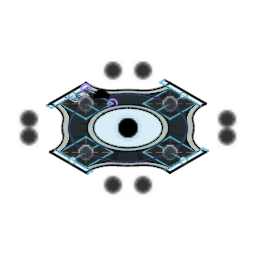
_Round About - Ruby.f2236e12-3166-4e72-b55a-dd2a6dc33c33 (Autodesk Fusion 360 design; units mm, degrees)
Autodesk Fusion 360 part; units mm, degrees
sketch "Sketch1" plane through (0, 0, 0) normal (0, 0, 1) x (1, 0, 0)
  circle A0 centre (0, 0) radius 660.4
  line L0 (660.4, 0) -> (1270, 0)
  line L1 (0, -660.4) -> (0, -1270)
  line L2 (-660.4, 0) -> (-1269.999981, 0)
  line L3 (0, 660.4) -> (0, 1270)
  circle A1 centre (0, 0) radius 965.2
  line L4 (1269.999981, 304.8) -> (660.400019, 304.8)
  line L5 (660.400019, 304.8) -> (660.400019, -304.8)
  line L6 (660.400019, -304.8) -> (1269.999981, -304.8)
  line L7 (1269.999981, -304.8) -> (1269.999981, 304.8)
  line L8 (1269.999981, 304.8) -> (660.400019, -304.8) construction
  line L9 (660.400019, 304.8) -> (1269.999981, -304.8) construction
  line L10 (304.8, 1270) -> (-304.8, 1270)
  line L11 (-304.8, 1270) -> (-304.8, 660.4)
  line L12 (-304.8, 660.4) -> (304.8, 660.4)
  line L13 (304.8, 660.4) -> (304.8, 1270)
  line L14 (304.8, 1270) -> (-304.8, 660.4) construction
  line L15 (-304.8, 1270) -> (304.8, 660.4) construction
  line L16 (-660.39999, 304.8) -> (-1269.99999, 304.8)
  line L17 (-1269.99999, 304.8) -> (-1269.99999, -304.8)
  line L18 (-1269.99999, -304.8) -> (-660.39999, -304.8)
  line L19 (-660.39999, -304.8) -> (-660.39999, 304.8)
  line L20 (-660.39999, 304.8) -> (-1269.99999, -304.8) construction
  line L21 (-1269.99999, 304.8) -> (-660.39999, -304.8) construction
  line L22 (304.8, -660.4) -> (-304.8, -660.4)
  line L23 (-304.8, -660.4) -> (-304.8, -1270)
  line L24 (-304.8, -1270) -> (304.8, -1270)
  line L25 (304.8, -1270) -> (304.8, -660.4)
  line L26 (304.8, -660.4) -> (-304.8, -1270) construction
  line L27 (-304.8, -660.4) -> (304.8, -1270) construction
  point P0 (965.2, 0)
  point P1 (0, 965.2)
  point P2 (-965.19999, 0)
  point P3 (0, -965.2)
  dimension "d1" = 1320.8
  dimension "d2" = 609.6
  dimension "d3" = 609.6
  dimension "d4" = 609.6
  dimension "d5" = 304.8
  dimension "d6" = 609.6
  dimension "d7" = 609.6
  dimension "d8" = 609.6
  dimension "d9" = 609.6
  dimension "d10" = 609.6
  dimension "d11" = 609.6
  dimension "d12" = 609.6
  constraint coincident A0.centre A1.centre
  constraint coincident A0 L0.start
  constraint horizontal L0
  constraint coincident A0 L1.start
  constraint vertical L1
  constraint coincident A0 L2.start
  constraint horizontal L2
  constraint coincident A0 L3.start
  constraint vertical L3
  constraint horizontal L4
  constraint perpendicular L4 L5
  constraint parallel L4 L6
  constraint parallel L5 L7
  constraint coincident L8 P0
  constraint coincident L9 P0
  constraint midpoint L0 P0
  constraint horizontal L10
  constraint perpendicular L10 L11
  constraint parallel L10 L12
  constraint parallel L11 L13
  constraint coincident L14 P1
  constraint coincident L15 P1
  constraint midpoint L3 P1
  constraint horizontal L16
  constraint perpendicular L16 L17
  constraint parallel L16 L18
  constraint parallel L17 L19
  constraint horizontal L22
  constraint perpendicular L22 L23
  constraint parallel L22 L24
  constraint parallel L23 L25
  constraint coincident L26 P3
  constraint coincident L27 P3
  constraint midpoint L1 P3
  measures "d1" diameter of A0
  measures "d2" distance of L0.start L0.end
  measures "d3" distance of L1.start L1.end
  measures "d4" distance of L3.start L3.end
  measures "d7" distance of L11.end L12.end
  measures "d8" distance of L10.end L11.end
  measures "d11" distance of L23.end L24.end
  measures "d12" distance of L22.end L23.end
extrude "Extrude1" add sketch "Sketch1" along normal blind 6.35 contours A0 A1 L5 L6 L22 L25 | L0 A1 L4 L5 | A0 A1 L4 L5 L12 L13 | L0 A1 L5 L6 | L3 A1 L11 L12 | A0 A1 L11 L12 L16 L19 | L3 A1 L12 L13 | A0 A1 L18 L19 L22 L23 | L1 A1 L22 L25 | L1 A1 L22 L23 | L2 A1 L18 L19 | L2 A1 L16 L19 picked at (676.405382, -534.145656) picked at (754.647884, 169.987105) picked at (676.405382, 534.145656) picked at (754.647877, -169.987105) picked at (-169.987105, 754.647871) picked at (-676.405382, 534.145656) picked at (169.987105, 754.647871) picked at (-676.405382, -534.145656) picked at (169.987105, -754.647871) picked at (-169.987105, -754.647871) picked at (-754.647865, -169.987105) picked at (-754.647868, 169.987105) makes body 1
extrude "Extrude2" add sketch "Sketch1" along normal blind 6.35 contours L0 A1 L4 L7 | L0 A1 L6 L7 | L3 A1 L10 L11 | L3 A1 L10 L13 | L1 A1 L24 L25 | L1 A1 L23 L24 | L2 A1 L17 L18 | L2 A1 L16 L17 picked at (1166.556681, 135.990587) picked at (1166.556675, -135.990587) picked at (-135.990587, 1166.556687) picked at (135.990587, 1166.556687) picked at (135.990587, -1166.556687) picked at (-135.990587, -1166.556687) picked at (-1166.556678, -135.990587) picked at (-1166.556681, 135.990587) bodies 1
fillet "Fillet1" radius 660.4 1 edges at (-915.810024, -304.8, 3.175) on bodies 1
fillet "Fillet2" radius 660.4 1 edges at (-304.8, -915.810024, 3.175) on bodies 1
fillet "Fillet3" radius 660.4 1 edges at (304.8, -915.810024, 3.175) on bodies 1
fillet "Fillet4" radius 660.4 1 edges at (915.810024, -304.8, 3.175) on bodies 1
fillet "Fillet5" radius 660.4 1 edges at (915.810024, 304.8, 3.175) on bodies 1
fillet "Fillet6" radius 660.4 1 edges at (304.8, 915.810024, 3.175) on bodies 1
fillet "Fillet7" radius 660.4 1 edges at (-304.8, 915.810024, 3.175) on bodies 1
fillet "Fillet8" radius 660.4 1 edges at (-915.810024, 304.8, 3.175) on bodies 1
sketch "Sketch2" plane through (0, 0, 6.35) normal (0, 0, 1) x (-1, 0, 0)
  arc A0 (572.40726, -777.149258) -> (777.149258, -572.40726) centre (0, 0) ccw
  arc A1 (1269.99999, -304.8) -> (777.149258, -572.40726) centre (1308.882961, -964.054332) ccw
  line L0 (1269.99999, -304.8) -> (1269.99999, 304.8)
  arc A2 (777.149258, 572.40726) -> (1269.99999, 304.8) centre (1308.882961, 964.054332) ccw
  arc A3 (777.149258, 572.40726) -> (572.40726, 777.149258) centre (0, 0) ccw
  arc A4 (304.8, 1270) -> (572.40726, 777.149258) centre (964.054333, 1308.88296) ccw
  line L1 (304.8, 1270) -> (-304.8, 1270)
  arc A5 (-572.40726, 777.149258) -> (-304.8, 1270) centre (-964.054333, 1308.88296) ccw
  arc A6 (-572.40726, 777.149258) -> (-777.149258, 572.407259) centre (0, 0) ccw
  arc A7 (-1269.999981, 304.8) -> (-777.149258, 572.407259) centre (-1308.882961, 964.054332) ccw
  line L2 (-1269.999981, 304.8) -> (-1269.999981, -304.8)
  arc A8 (-777.149258, -572.407259) -> (-1269.999981, -304.8) centre (-1308.882961, -964.054332) ccw
  arc A9 (-777.149258, -572.407259) -> (-572.40726, -777.149258) centre (0, 0) ccw
  arc A10 (-304.8, -1270) -> (-572.40726, -777.149258) centre (-964.054333, -1308.88296) ccw
  line L3 (-304.8, -1270) -> (304.8, -1270)
  arc A11 (572.40726, -777.149258) -> (304.8, -1270) centre (964.054333, -1308.88296) ccw
  arc A12 (660.4, 0) -> (660.399997, -0.064797) centre (0, 0) ccw
  line L4 (660.4, 0) -> (660.399997, -0.064797)
  line L5 (558.8, 0.002492) -> (558.799997, -0.057321)
  arc A13 (558.8, 0.002492) -> (558.799997, -0.057321) centre (0, 0) ccw
  line L6 (-1371.599981, 408.785014) -> (-1371.599981, -408.785014)
  arc A14 (-858.954443, -632.660655) -> (-1371.599981, -408.785014) centre (-1308.882961, -964.054332) ccw
  arc A15 (-858.954443, -632.660655) -> (-632.660656, -858.954443) centre (0, 0) ccw
  arc A16 (-408.785017, -1371.6) -> (-632.660656, -858.954443) centre (-964.054333, -1308.88296) ccw
  line L7 (-408.785017, -1371.6) -> (408.785017, -1371.6)
  arc A17 (632.660656, -858.954443) -> (408.785017, -1371.6) centre (964.054333, -1308.88296) ccw
  arc A18 (632.660656, -858.954443) -> (858.954443, -632.660656) centre (0, 0) ccw
  arc A19 (1371.59999, -408.785016) -> (858.954443, -632.660656) centre (1308.882961, -964.054332) ccw
  line L8 (1371.59999, -408.785016) -> (1371.59999, 408.785016)
  arc A20 (858.954443, 632.660656) -> (1371.59999, 408.785016) centre (1308.882961, 964.054332) ccw
  arc A21 (858.954443, 632.660656) -> (632.660656, 858.954443) centre (0, 0) ccw
  arc A22 (408.785017, 1371.6) -> (632.660656, 858.954443) centre (964.054333, 1308.88296) ccw
  line L9 (408.785017, 1371.6) -> (-408.785017, 1371.6)
  arc A23 (-632.660656, 858.954443) -> (-408.785017, 1371.6) centre (-964.054333, 1308.88296) ccw
  arc A24 (-632.660656, 858.954443) -> (-858.954443, 632.660655) centre (0, 0) ccw
  arc A25 (-1371.599981, 408.785014) -> (-858.954443, 632.660655) centre (-1308.882961, 964.054332) ccw
  line L10 (-1371.599981, 408.785014) -> (-1269.999981, 408.785014)
  line L11 (-1269.999981, 408.785014) -> (-1269.999981, -457.199993)
  line L12 (-1269.999981, -457.199993) -> (-1371.599981, -457.199993)
  line L13 (-1371.599981, -457.199993) -> (-1371.599981, 408.785014)
  line L14 (-408.785017, -1371.6) -> (533.399992, -1371.6)
  line L15 (533.399992, -1371.6) -> (533.399992, -1269.999981)
  line L16 (533.399992, -1269.999981) -> (-408.785017, -1269.999981)
  line L17 (-408.785017, -1269.999981) -> (-408.785017, -1371.6)
  line L18 (1371.59999, -408.785016) -> (1269.999981, -408.785016)
  line L19 (1269.999981, -408.785016) -> (1269.999981, 482.599993)
  line L20 (1269.999981, 482.599993) -> (1371.59999, 482.599993)
  line L21 (1371.59999, 482.599993) -> (1371.59999, -408.785016)
  line L22 (408.785017, 1371.6) -> (-447.666394, 1371.6)
  line L23 (-447.666394, 1371.6) -> (-447.666394, 1270)
  line L24 (-447.666394, 1270) -> (408.785017, 1270)
  line L25 (408.785017, 1270) -> (408.785017, 1371.6)
  line L26 (660.39999, -304.8, -6.35) -> (1269.99999, -304.8, -6.35)
  circle A26 through (965.2, 0, -6.35) (-482.6, 835.88772, -6.35) (-482.6, -835.88772, -6.35)
  point P0 (915.810024, -304.8)
  dimension "d33" = -101.6
  dimension "d34" = -101.6
  constraint horizontal L10
  constraint vertical L11
  constraint horizontal L12
  constraint vertical L13
  constraint horizontal L14
  constraint vertical L15
  constraint horizontal L16
  constraint vertical L17
  constraint horizontal L18
  constraint vertical L19
  constraint horizontal L20
  constraint vertical L21
  constraint horizontal L22
  constraint vertical L23
  constraint horizontal L24
  constraint vertical L25
extrude "Extrude1'" add sketch "Sketch2" against normal blind 6.35 separate body contours A0 A1 A11 A17 A18 A19 L16 L19 | A8 A9 A10 A14 A15 A16 L11 L16 | A2 A3 A4 A20 A21 A22 L19 L24 | A5 A6 A7 A23 A24 A25 L11 L24 | A12 L4 picked at (809.112672, -640.205668) picked at (-665.203767, -788.689142) picked at (640.205668, 809.112672) picked at (-809.112673, 640.205667) picked at (624.074703, 32.809493) makes body 2 at (-809.112672, 640.205668, 6.35) makes body 3 at (-640.205668, -809.112672, 6.35) makes body 4 at (665.203767, 788.689142, 6.35) makes body 5 at (809.112673, -640.205667, 6.35) makes body 6 at (-624.074703, -32.809493, 6.35) in component "Round About"
copy_body "CutPasteBodies1" bodies 1 removing the originals makes body 7 in component "Round About"
component "Round About" placed x (1, 0, 0) y (0, 1, 0) z (0, 0, 1) at (0, 0, 0)
